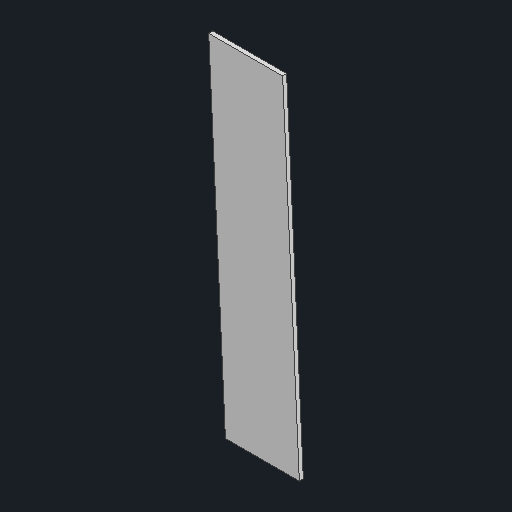
# Autodesk Inventor part: sponson_indent
Saved by Autodesk Inventor 2023 (Build 270158030, 158C)
## iProperties
Created: 2022-03-24
Part Number: sponson_indent
Material: Generic
Document SubType Name: Modeling
Designer: kardo
Density: 1 g/cm^3
Appearance: Default
Author: kardo
Autodesk Inventor part; units mm, degrees
ref_plane "YZ Plane" through (0, 0, 0) normal (1, 0, 0) x (0, 1, 0)
ref_plane "XZ Plane" through (0, 0, 0) normal (0, 1, 0) x (-1, 0, 0)
ref_plane "XY Plane" through (0, 0, 0) normal (0, 0, 1) x (1, 0, 0)
derived "parameters_frame.ipt"
derived "surface_body.ipt"
sketch "sk_long_outer" plane through (0, 0, 0) normal (1, 0, 0) x (0, 1, 0)
  line L0 (-363, 107.6209) -> (-363, -224.5198) construction
  line L1 (237, 107.6209) -> (237, -224.5198) construction
  line L2 (-483, 54.4) -> (357, 54.4) construction
  line L3 (-483, 0) -> (357, 0) construction
  line L4 (0, 107.6209) -> (0, -224.5198) construction
  line L5 (0, 6.528) -> (-363, 11.424)
  line L6 (-363, 11.424) -> (-363, 39.712)
  line L7 (-363, 39.712) -> (0, 54.4)
  line L8 (0, 54.4) -> (237, 36.448)
  line L9 (0, 0) -> (111.39, 7.7891)
  line L10 (111.39, 7.7891) -> (237, 36.448)
  line L11 (0, 6.528) -> (0, 0)
  line L12 (0, 6.528) -> (111.1168, 11.6964)
  line L13 (111.1168, 11.6964) -> (111.39, 7.7891)
sketch "sk_cross" plane through (0, 0, 0) normal (0, 1, 0) x (-1, 0, 0)
  line L0 (0, -224.5198) -> (0, 107.6209) construction
  line L1 (-156, -224.5198) -> (-156, 107.6209) construction
  line L2 (156, -224.5198) -> (156, 107.6209)
  line L3 (-188.7979, 0) -> (31.4663, 0) construction
  line L4 (-188.7979, 54.4) -> (31.4663, 54.4) construction
  line L5 (-81.12, -224.5198) -> (-81.12, 107.6209) construction
  line L6 (-54.6, -224.5198) -> (-54.6, 107.6209) construction
  line L7 (-34.32, -224.5198) -> (-34.32, 107.6209) construction
  line L8 (0, 54.4) -> (-54.6, 54.4)
  line L9 (-54.6, 54.4) -> (-81.12, 52.8758)
  line L10 (-81.12, 0) -> (-81.12, 52.8758)
  line L11 (-81.12, 6.528) -> (-112.356, 43.7537)
  line L12 (-156, 31.008) -> (-126.048, 0)
  line L13 (-126.048, 0) -> (-81.12, 0)
  line L14 (-81.12, 52.8758) -> (-156, 31.008)
  arc A0 (-54.6, 54.4) -> (-156, 31.008) centre (-54.6, -177.0711) ccw construction
  line L15 (-81.12, 6.528) -> (-103.584, 6.528)
  line L16 (-103.584, 6.528) -> (-103.584, 0)
  point P0 (0, 0)
ref_plane "plane_tunnel_right" through (81.12, 0, 0) normal (1, 0, 0) x (0, 1, 0)
sketch "sk_profile" plane through (81.12, 0, 0) normal (1, 0, 0) x (0, 1, 0)
  line L0 (0, 6.528) -> (109.1189, 11.6035)
  line L1 (109.1189, 11.6035) -> (111.1168, 11.6964) construction
  point P0 (0, 0)
  dimension "d2" = 2
  constraints: 4 end point, 1 collinear
  measures "d2" distance of L0.end L1.end
surface extrude "surface" sketch "sk_profile" along normal up to surface (22.464 mm away) shown no curves L0
thicken "thicken" operation new thickness 1.2 both sides no extend neighbours no toward (0, -0.0464631, 0.99892) faces at (96.096, 36.373, 8.2198)
equation "\"d2\" = bulkhead_thickness"
equation "\"d5\" = shell_thickness"
equation "\"d6\" = shell_thickness"
equation "\"bulkhead_thickness\" = 2"
equation "\"shell_thickness\" = 1.2"
body "Solid1"
body "Srf1"
